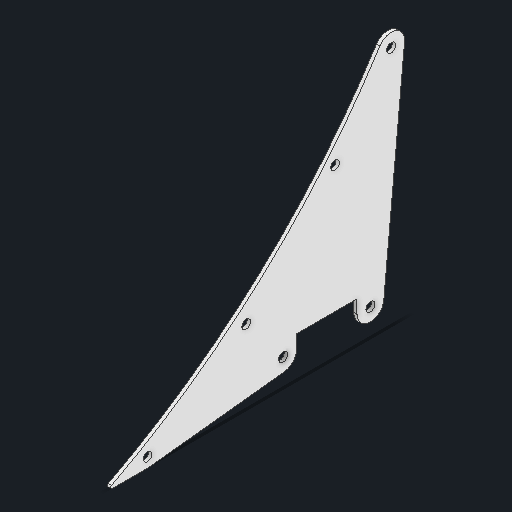
# Autodesk Inventor part: Ramp V2
Saved by Autodesk Inventor 2025.1 (Build 291241000, 241)
## iProperties
Created: 2024-10-13
Part Number: Ramp V2
Material: Acetal Resin, White
Document SubType Name: Sheet Metal
Designer: Averey Ku
Density: 1.425 g/cm^3
Appearance: Smooth - White
Mass: 12.8393 g
Surface Area: 122.133 cm^2
Volume: 9.01001 cm^3
Flat Pattern Width: 12.3031 cm
Flat Pattern Length: 14.8051 cm
Flat Pattern Area: 182.149 cm^2
Sheet Metal Rule: Default_mm
Sheet Metal Width: 4.844 in
Sheet Metal Length: 5.829 in
Sheet Metal Area: 28.233 in^2
Author: Averey Ku
Autodesk Inventor part; units mm, degrees
ref_plane "YZ Plane" through (0, 0, 0) normal (1, 0, 0) x (0, 1, 0)
ref_plane "XZ Plane" through (0, 0, 0) normal (0, 1, 0) x (-1, 0, 0)
ref_plane "XY Plane" through (0, 0, 0) normal (0, 0, 1) x (1, 0, 0)
sketch "main" plane through (0, 0, 0) normal (0, 0, 1) x (1, 0, 0)
  circle A0 centre (-198.1135, 49.9495) radius 2.1844
  circle A1 centre (-97.0008, -1.1659) radius 2.1
  arc A2 (-97.6159, -7.486) -> (-93.6005, 4.197) centre (-97.0008, -1.1659) ccw
  arc A3 (-204.4247, 49.249) -> (-198.1135, 43.5995) centre (-198.1135, 49.9495) ccw
  arc A4 (-210.0929, 131.0519) -> (-93.6005, 4.197) centre (83.8489, 284.0666) ccw
  circle A5 centre (-206.8262, 114.0524) radius 2.0828
  arc A6 (-210.0929, 131.0519) -> (-211.5759, 130.5326) centre (-210.797, 130.6854) ccw
  circle A7 centre (-131.7625, 25.4) radius 2.0828
  line L0 (-198.7286, 2.3544) -> (-97.6159, -7.486)
  circle A8 centre (-198.1135, 8.6745) radius 2.1848
  arc A9 (-198.1135, 15.0245) -> (-198.7286, 2.3544) centre (-198.1135, 8.6745) ccw
  line L1 (-211.5828, 130.7972) -> (-211.5828, 113.8158)
  arc A10 (-211.5828, 114.289) -> (-211.5596, 113.527) centre (-206.8262, 114.0524) ccw
  line L2 (-211.5596, 113.527) -> (-204.4247, 49.249)
  circle A11 centre (-175.8885, 67.412) radius 2.0955
  point P0 (1.1251, 9.7944)
  point P1 (-211.9386, 134.6509)
  point P2 (-191.7635, 49.9495)
  dimension "d7" = 12.7
  dimension "d8" = 4.1656
  dimension "d9" = 6.35
  dimension "d13" = 4.1656
  dimension "d20" = 0
  dimension "d21" = 6.35
  dimension "d26" = 9.525
  dimension "d27" = 4.191
  measures "d7" diameter of A3
  measures "d8" diameter of A5
  measures "d9" radius of A2
  measures "d13" diameter of A7
  measures "d20" vertical distance of point (-191.763, 49.95) A0.centre
  measures "d21" distance of point (-191.763, 49.95) A0.centre
  measures "d26" diameter of A10
  measures "d27" diameter of A11
sketch "Sketch1" plane through (0, 0, 0) normal (1, 0, 0) x (0, 1, 0)
  line L0 (6.35, -9.525) -> (6.35, -7.9375) projected
  line L1 (6.35, -6.35) -> (6.35, -34.925)
  line L2 (0, -6.35) -> (6.35, -6.35)
  line L3 (0, -34.925) -> (6.35, -34.925)
  circle A0 centre (101.1127, -51.1154) radius 2.1844 projected
  circle A1 centre (0, 0) radius 2.1844
  circle A2 centre (101.1127, -51.1154) radius 2.1
  arc A3 (100.4976, -57.4355) -> (104.5129, -45.7525) centre (101.1127, -51.1154) ccw
  arc A4 (-6.3112, -0.7006) -> (0, -6.35) centre (0, 0) ccw
  arc A5 (-11.9794, 81.1024) -> (104.5129, -45.7525) centre (281.9624, 234.117) ccw
  circle A6 centre (-8.7127, 64.1028) radius 2.0828
  arc A7 (-11.9794, 81.1024) -> (-13.4624, 80.5831) centre (-12.6835, 80.7359) ccw
  circle A8 centre (66.351, -24.5495) radius 2.0828
  line L4 (-0.6151, -47.5951) -> (100.4976, -57.4355)
  circle A9 centre (0, -41.275) radius 2.1848
  arc A10 (0, -34.925) -> (-0.6151, -47.5951) centre (0, -41.275) ccw
  line L5 (-13.4693, 80.8476) -> (-13.4693, 63.8663)
  arc A11 (-13.4693, 64.3394) -> (-13.4461, 63.5774) centre (-8.7127, 64.1028) ccw
  line L6 (-13.4461, 63.5774) -> (-6.3112, -0.7006)
  circle A12 centre (22.225, 17.4625) radius 2.0955
  point P0 (0, -6.35)
  point P1 (0, -34.925)
  constraints: 6 end point, 1 horizontal, 3 other
extrude "Extrusion1" add sketch "Sketch1" along normal blind 1.5875 contours L0 L1 L2 A4 L6 A11 L5 A7 A5 A3 L4 A10 L3
equation "\"BendRadius\" = Thickness"
equation "\"BendReliefWidth\" = Thickness"
equation "\"BendReliefDepth\" = 0.5 * Thickness"
equation "\"CornerReliefSize\" = 4 * Thickness"
equation "\"MinimumRemnant\" = 2 * Thickness"
equation "\"TransitionRadius\" = BendRadius"
equation "\"JacobiRadiusSize\" = BendRadius"
equation "\"GapSize\" = Thickness"
equation "\"Thickness\" = 1.5875"
body "Solid1"
